Autodesk Fusion 360 part; units mm, degrees
(part 30 of 40)
  line L6927 (266.9246, 183.2292) -> (267.0281, 183.3491) construction
  line L6928 (267.0281, 183.3491) -> (267.1308, 183.47) construction
  line L6929 (267.1308, 183.47) -> (267.2327, 183.5919) construction
  line L6930 (267.2327, 183.5919) -> (267.3337, 183.7148) construction
  line L6931 (267.3337, 183.7148) -> (267.434, 183.8386) construction
  line L6932 (267.434, 183.8386) -> (267.5335, 183.9633) construction
  line L6933 (267.5335, 183.9633) -> (267.6323, 184.0888) construction
  line L6934 (267.6323, 184.0888) -> (267.7304, 184.2151) construction
  line L6935 (267.7304, 184.2151) -> (267.8277, 184.3423) construction
  line L6936 (267.8277, 184.3423) -> (267.9243, 184.4703) construction
  line L6937 (267.9243, 184.4703) -> (268.0201, 184.5991) construction
  line L6938 (268.0201, 184.5991) -> (268.1152, 184.7288) construction
  line L6939 (268.1152, 184.7288) -> (268.2096, 184.8592) construction
  line L6940 (268.2096, 184.8592) -> (268.3032, 184.9905) construction
  line L6941 (268.3032, 184.9905) -> (268.3962, 185.1224) construction
  line L6942 (268.3962, 185.1224) -> (268.4884, 185.2552) construction
  line L6943 (268.4884, 185.2552) -> (268.58, 185.3886) construction
  line L6944 (268.58, 185.3886) -> (268.6708, 185.5228) construction
  line L6945 (268.6708, 185.5228) -> (268.761, 185.6577) construction
  line L6946 (268.761, 185.6577) -> (268.8505, 185.7933) construction
  line L6947 (268.8505, 185.7933) -> (268.9393, 185.9295) construction
  line L6948 (268.9393, 185.9295) -> (269.0275, 186.0665) construction
  line L6949 (269.0275, 186.0665) -> (269.1149, 186.2042) construction
  line L6950 (269.1149, 186.2042) -> (269.2017, 186.3425) construction
  line L6951 (269.2017, 186.3425) -> (269.2878, 186.4815) construction
  line L6952 (269.2878, 186.4815) -> (269.3733, 186.6211) construction
  line L6953 (269.3733, 186.6211) -> (269.4581, 186.7614) construction
  line L6954 (269.4581, 186.7614) -> (269.5422, 186.9023) construction
  line L6955 (269.5422, 186.9023) -> (269.6257, 187.0438) construction
  line L6956 (269.6257, 187.0438) -> (269.7085, 187.186) construction
  line L6957 (269.7085, 187.186) -> (269.7907, 187.3288) construction
  line L6958 (269.7907, 187.3288) -> (269.8723, 187.4721) construction
  line L6959 (269.8723, 187.4721) -> (269.9532, 187.6161) construction
  line L6960 (269.9532, 187.6161) -> (270.0334, 187.7607) construction
  line L6961 (270.0334, 187.7607) -> (270.113, 187.9058) construction
  line L6962 (270.113, 187.9058) -> (270.192, 188.0515) construction
  line L6963 (270.192, 188.0515) -> (270.2703, 188.1978) construction
  line L6964 (270.2703, 188.1978) -> (270.348, 188.3447) construction
  line L6965 (270.348, 188.3447) -> (270.4251, 188.4921) construction
  line L6966 (270.4251, 188.4921) -> (270.5015, 188.6401) construction
  line L6967 (270.5015, 188.6401) -> (270.5773, 188.7886) construction
  line L6968 (270.5773, 188.7886) -> (270.6525, 188.9377) construction
  line L6969 (270.6525, 188.9377) -> (270.727, 189.0873) construction
  line L6970 (270.727, 189.0873) -> (270.801, 189.2374) construction
  line L6971 (270.801, 189.2374) -> (270.8743, 189.3881) construction
  line L6972 (270.8743, 189.3881) -> (270.9469, 189.5393) construction
  line L6973 (270.9469, 189.5393) -> (271.019, 189.6909) construction
  line L6974 (271.019, 189.6909) -> (271.0904, 189.8431) construction
  line L6975 (271.0904, 189.8431) -> (271.1471, 189.9653) construction
  line L6976 (271.1471, 189.9653) -> (271.1893, 190.0572) construction
  line L6977 (271.1893, 190.0572) -> (271.2173, 190.1185) construction
  line L6978 (271.2173, 190.1185) -> (271.2313, 190.1492) construction
  arc A182 (271.2762, 144.4572) -> (269.1057, 142.7194) centre (271.0895, 142.4659) ccw
  spline S93 degree 5 poles (264.6423, 118.8885) (264.6688, 118.8728) (264.7215, 118.8406) (264.7992, 118.7903) (264.9001, 118.7193) (265.0226, 118.6252) (265.1426, 118.5273) (265.2609, 118.4271) (265.3784, 118.3256) (265.4954, 118.2233) (265.6117, 118.12) (265.7271, 118.0156) (265.8414, 117.9097) (265.9544, 117.8019) (266.066, 117.6923) (266.1764, 117.581) (266.2857, 117.4684) (266.3942, 117.3545) (266.5018, 117.2397) (266.6087, 117.124) (266.7148, 117.0073) (266.8201, 116.8895) (266.9246, 116.7708) (267.0281, 116.6509) (267.1308, 116.53) (267.2327, 116.4081) (267.3337, 116.2852) (267.434, 116.1614) (267.5335, 116.0367) (267.6323, 115.9112) (267.7304, 115.7849) (267.8277, 115.6577) (267.9243, 115.5297) (268.0201, 115.4009) (268.1152, 115.2712) (268.2096, 115.1408) (268.3032, 115.0095) (268.3962, 114.8776) (268.4884, 114.7448) (268.58, 114.6114) (268.6708, 114.4772) (268.761, 114.3423) (268.8505, 114.2067) (268.9393, 114.0705) (269.0275, 113.9335) (269.1149, 113.7958) (269.2017, 113.6575) (269.2878, 113.5185) (269.3733, 113.3789) (269.4581, 113.2386) (269.5422, 113.0977) (269.6257, 112.9562) (269.7085, 112.814) (269.7907, 112.6712) (269.8723, 112.5279) (269.9532, 112.3839) (270.0334, 112.2393) (270.113, 112.0942) (270.192, 111.9485) (270.2703, 111.8022) (270.348, 111.6553) (270.4251, 111.5079) (270.5015, 111.3599) (270.5773, 111.2114) (270.6525, 111.0623) (270.727, 110.9127) (270.801, 110.7626) (270.8743, 110.6119) (270.9469, 110.4607) (271.019, 110.3091) (271.0904, 110.1569) (271.1471, 110.0347) (271.1893, 109.9428) (271.2173, 109.8815) (271.2313, 109.8508) knots 0 0 0 0 0 0 0.01428571 0.02857143 0.04285714 0.05714286 0.07142857 0.08571429 0.1 0.11428571 0.12857143 0.14285714 0.15714286 0.17142857 0.18571429 0.2 0.21428571 0.22857143 0.24285714 0.25714286 0.27142857 0.28571429 0.3 0.31428571 0.32857143 0.34285714 0.35714286 0.37142857 0.38571429 0.4 0.41428571 0.42857143 0.44285714 0.45714286 0.47142857 0.48571429 0.5 0.51428571 0.52857143 0.54285714 0.55714286 0.57142857 0.58571429 0.6 0.61428571 0.62857143 0.64285714 0.65714286 0.67142857 0.68571429 0.7 0.71428571 0.72857143 0.74285714 0.75714286 0.77142857 0.78571429 0.8 0.81428571 0.82857143 0.84285714 0.85714286 0.87142857 0.88571429 0.9 0.91428571 0.92857143 0.94285714 0.95714286 0.97142857 0.98571429 1 1 1 1 1 1
  line L6979 (264.6423, 118.8885) -> (264.6688, 118.8728) construction
  line L6980 (264.6688, 118.8728) -> (264.7215, 118.8406) construction
  line L6981 (264.7215, 118.8406) -> (264.7992, 118.7903) construction
  line L6982 (264.7992, 118.7903) -> (264.9001, 118.7193) construction
  line L6983 (264.9001, 118.7193) -> (265.0226, 118.6252) construction
  line L6984 (265.0226, 118.6252) -> (265.1426, 118.5273) construction
  line L6985 (265.1426, 118.5273) -> (265.2609, 118.4271) construction
  line L6986 (265.2609, 118.4271) -> (265.3784, 118.3256) construction
  line L6987 (265.3784, 118.3256) -> (265.4954, 118.2233) construction
  line L6988 (265.4954, 118.2233) -> (265.6117, 118.12) construction
  line L6989 (265.6117, 118.12) -> (265.7271, 118.0156) construction
  line L6990 (265.7271, 118.0156) -> (265.8414, 117.9097) construction
  line L6991 (265.8414, 117.9097) -> (265.9544, 117.8019) construction
  line L6992 (265.9544, 117.8019) -> (266.066, 117.6923) construction
  line L6993 (266.066, 117.6923) -> (266.1764, 117.581) construction
  line L6994 (266.1764, 117.581) -> (266.2857, 117.4684) construction
  line L6995 (266.2857, 117.4684) -> (266.3942, 117.3545) construction
  line L6996 (266.3942, 117.3545) -> (266.5018, 117.2397) construction
  line L6997 (266.5018, 117.2397) -> (266.6087, 117.124) construction
  line L6998 (266.6087, 117.124) -> (266.7148, 117.0073) construction
  line L6999 (266.7148, 117.0073) -> (266.8201, 116.8895) construction
  line L7000 (266.8201, 116.8895) -> (266.9246, 116.7708) construction
  line L7001 (266.9246, 116.7708) -> (267.0281, 116.6509) construction
  line L7002 (267.0281, 116.6509) -> (267.1308, 116.53) construction
  line L7003 (267.1308, 116.53) -> (267.2327, 116.4081) construction
  line L7004 (267.2327, 116.4081) -> (267.3337, 116.2852) construction
  line L7005 (267.3337, 116.2852) -> (267.434, 116.1614) construction
  line L7006 (267.434, 116.1614) -> (267.5335, 116.0367) construction
  line L7007 (267.5335, 116.0367) -> (267.6323, 115.9112) construction
  line L7008 (267.6323, 115.9112) -> (267.7304, 115.7849) construction
  line L7009 (267.7304, 115.7849) -> (267.8277, 115.6577) construction
  line L7010 (267.8277, 115.6577) -> (267.9243, 115.5297) construction
  line L7011 (267.9243, 115.5297) -> (268.0201, 115.4009) construction
  line L7012 (268.0201, 115.4009) -> (268.1152, 115.2712) construction
  line L7013 (268.1152, 115.2712) -> (268.2096, 115.1408) construction
  line L7014 (268.2096, 115.1408) -> (268.3032, 115.0095) construction
  line L7015 (268.3032, 115.0095) -> (268.3962, 114.8776) construction
  line L7016 (268.3962, 114.8776) -> (268.4884, 114.7448) construction
  line L7017 (268.4884, 114.7448) -> (268.58, 114.6114) construction
  line L7018 (268.58, 114.6114) -> (268.6708, 114.4772) construction
  line L7019 (268.6708, 114.4772) -> (268.761, 114.3423) construction
  line L7020 (268.761, 114.3423) -> (268.8505, 114.2067) construction
  line L7021 (268.8505, 114.2067) -> (268.9393, 114.0705) construction
  line L7022 (268.9393, 114.0705) -> (269.0275, 113.9335) construction
  line L7023 (269.0275, 113.9335) -> (269.1149, 113.7958) construction
  line L7024 (269.1149, 113.7958) -> (269.2017, 113.6575) construction
  line L7025 (269.2017, 113.6575) -> (269.2878, 113.5185) construction
  line L7026 (269.2878, 113.5185) -> (269.3733, 113.3789) construction
  line L7027 (269.3733, 113.3789) -> (269.4581, 113.2386) construction
  line L7028 (269.4581, 113.2386) -> (269.5422, 113.0977) construction
  line L7029 (269.5422, 113.0977) -> (269.6257, 112.9562) construction
  line L7030 (269.6257, 112.9562) -> (269.7085, 112.814) construction
  line L7031 (269.7085, 112.814) -> (269.7907, 112.6712) construction
  line L7032 (269.7907, 112.6712) -> (269.8723, 112.5279) construction
  line L7033 (269.8723, 112.5279) -> (269.9532, 112.3839) construction
  line L7034 (269.9532, 112.3839) -> (270.0334, 112.2393) construction
  line L7035 (270.0334, 112.2393) -> (270.113, 112.0942) construction
  line L7036 (270.113, 112.0942) -> (270.192, 111.9485) construction
  line L7037 (270.192, 111.9485) -> (270.2703, 111.8022) construction
  line L7038 (270.2703, 111.8022) -> (270.348, 111.6553) construction
  line L7039 (270.348, 111.6553) -> (270.4251, 111.5079) construction
  line L7040 (270.4251, 111.5079) -> (270.5015, 111.3599) construction
  line L7041 (270.5015, 111.3599) -> (270.5773, 111.2114) construction
  line L7042 (270.5773, 111.2114) -> (270.6525, 111.0623) construction
  line L7043 (270.6525, 111.0623) -> (270.727, 110.9127) construction
  line L7044 (270.727, 110.9127) -> (270.801, 110.7626) construction
  line L7045 (270.801, 110.7626) -> (270.8743, 110.6119) construction
  line L7046 (270.8743, 110.6119) -> (270.9469, 110.4607) construction
  line L7047 (270.9469, 110.4607) -> (271.019, 110.3091) construction
  line L7048 (271.019, 110.3091) -> (271.0904, 110.1569) construction
  line L7049 (271.0904, 110.1569) -> (271.1471, 110.0347) construction
  line L7050 (271.1471, 110.0347) -> (271.1893, 109.9428) construction
  line L7051 (271.1893, 109.9428) -> (271.2173, 109.8815) construction
  line L7052 (271.2173, 109.8815) -> (271.2313, 109.8508) construction
  line L7053 (188.5839, 95.4634) -> (187.9372, 93.9655)
  line L7054 (161.0254, 180.2798) -> (159.6217, 181.1115)
  spline S94 degree 5 poles (151.3635, 155.6951) (151.3327, 155.6979) (151.2711, 155.7029) (151.1787, 155.7078) (151.0554, 155.7097) (150.901, 155.7056) (150.7464, 155.6969) (150.5917, 155.6854) (150.437, 155.6723) (150.2822, 155.6583) (150.1275, 155.6431) (149.9727, 155.6265) (149.818, 155.608) (149.6632, 155.5871) (149.5085, 155.5641) (149.3538, 155.539) (149.1991, 155.5121) (149.0445, 155.4838) (148.8899, 155.4542) (148.7354, 155.4233) (148.5809, 155.3913) (148.4265, 155.3579) (148.2722, 155.3232) (148.118, 155.2871) (147.9638, 155.2497) (147.8098, 155.2109) (147.6558, 155.1709) (147.5019, 155.1297) (147.3481, 155.0873) (147.1944, 155.0439) (147.0408, 154.9993) (146.8873, 154.9536) (146.734, 154.9068) (146.5807, 154.8589) (146.4276, 154.8099) (146.2746, 154.7599) (146.1217, 154.7087) (145.9689, 154.6566) (145.8162, 154.6035) (145.6637, 154.5493) (145.5114, 154.4942) (145.3591, 154.438) (145.207, 154.381) (145.055, 154.3229) (144.9032, 154.2639) (144.7516, 154.2039) (144.6, 154.143) (144.4487, 154.0812) (144.2975, 154.0185) (144.1464, 153.9548) (143.9955, 153.8903) (143.8448, 153.8249) (143.6942, 153.7585) (143.5438, 153.6913) (143.3936, 153.6233) (143.2435, 153.5543) (143.0936, 153.4846) (142.9439, 153.4139) (142.7944, 153.3425) (142.645, 153.2701) (142.4958, 153.197) (142.3468, 153.123) (142.198, 153.0482) (142.0494, 152.9726) (141.9009, 152.8962) (141.7527, 152.819) (141.6046, 152.741) (141.4568, 152.6622) (141.3091, 152.5826) (141.1617, 152.5023) (141.0144, 152.4211) (140.8968, 152.3556) (140.8086, 152.3061) (140.7499, 152.2729) (140.7205, 152.2563) knots 0 0 0 0 0 0 0.01428571 0.02857143 0.04285714 0.05714286 0.07142857 0.08571429 0.1 0.11428571 0.12857143 0.14285714 0.15714286 0.17142857 0.18571429 0.2 0.21428571 0.22857143 0.24285714 0.25714286 0.27142857 0.28571429 0.3 0.31428571 0.32857143 0.34285714 0.35714286 0.37142857 0.38571429 0.4 0.41428571 0.42857143 0.44285714 0.45714286 0.47142857 0.48571429 0.5 0.51428571 0.52857143 0.54285714 0.55714286 0.57142857 0.58571429 0.6 0.61428571 0.62857143 0.64285714 0.65714286 0.67142857 0.68571429 0.7 0.71428571 0.72857143 0.74285714 0.75714286 0.77142857 0.78571429 0.8 0.81428571 0.82857143 0.84285714 0.85714286 0.87142857 0.88571429 0.9 0.91428571 0.92857143 0.94285714 0.95714286 0.97142857 0.98571429 1 1 1 1 1 1
  line L7055 (151.3635, 155.6951) -> (151.3327, 155.6979) construction
  line L7056 (151.3327, 155.6979) -> (151.2711, 155.7029) construction
  line L7057 (151.2711, 155.7029) -> (151.1787, 155.7078) construction
  line L7058 (151.1787, 155.7078) -> (151.0554, 155.7097) construction
  line L7059 (151.0554, 155.7097) -> (150.901, 155.7056) construction
  line L7060 (150.901, 155.7056) -> (150.7464, 155.6969) construction
  line L7061 (150.7464, 155.6969) -> (150.5917, 155.6854) construction
  line L7062 (150.5917, 155.6854) -> (150.437, 155.6723) construction
  line L7063 (150.437, 155.6723) -> (150.2822, 155.6583) construction
  line L7064 (150.2822, 155.6583) -> (150.1275, 155.6431) construction
  line L7065 (150.1275, 155.6431) -> (149.9727, 155.6265) construction
  line L7066 (149.9727, 155.6265) -> (149.818, 155.608) construction
  line L7067 (149.818, 155.608) -> (149.6632, 155.5871) construction
  line L7068 (149.6632, 155.5871) -> (149.5085, 155.5641) construction
  line L7069 (149.5085, 155.5641) -> (149.3538, 155.539) construction
  line L7070 (149.3538, 155.539) -> (149.1991, 155.5121) construction
  line L7071 (149.1991, 155.5121) -> (149.0445, 155.4838) construction
  line L7072 (149.0445, 155.4838) -> (148.8899, 155.4542) construction
  line L7073 (148.8899, 155.4542) -> (148.7354, 155.4233) construction
  line L7074 (148.7354, 155.4233) -> (148.5809, 155.3913) construction
  line L7075 (148.5809, 155.3913) -> (148.4265, 155.3579) construction
  line L7076 (148.4265, 155.3579) -> (148.2722, 155.3232) construction
  line L7077 (148.2722, 155.3232) -> (148.118, 155.2871) construction
  line L7078 (148.118, 155.2871) -> (147.9638, 155.2497) construction
  line L7079 (147.9638, 155.2497) -> (147.8098, 155.2109) construction
  line L7080 (147.8098, 155.2109) -> (147.6558, 155.1709) construction
  line L7081 (147.6558, 155.1709) -> (147.5019, 155.1297) construction
  line L7082 (147.5019, 155.1297) -> (147.3481, 155.0873) construction
  line L7083 (147.3481, 155.0873) -> (147.1944, 155.0439) construction
  line L7084 (147.1944, 155.0439) -> (147.0408, 154.9993) construction
  line L7085 (147.0408, 154.9993) -> (146.8873, 154.9536) construction
  line L7086 (146.8873, 154.9536) -> (146.734, 154.9068) construction
  line L7087 (146.734, 154.9068) -> (146.5807, 154.8589) construction
  line L7088 (146.5807, 154.8589) -> (146.4276, 154.8099) construction
  line L7089 (146.4276, 154.8099) -> (146.2746, 154.7599) construction
  line L7090 (146.2746, 154.7599) -> (146.1217, 154.7087) construction
  line L7091 (146.1217, 154.7087) -> (145.9689, 154.6566) construction
  line L7092 (145.9689, 154.6566) -> (145.8162, 154.6035) construction
  line L7093 (145.8162, 154.6035) -> (145.6637, 154.5493) construction
  line L7094 (145.6637, 154.5493) -> (145.5114, 154.4942) construction
  line L7095 (145.5114, 154.4942) -> (145.3591, 154.438) construction
  line L7096 (145.3591, 154.438) -> (145.207, 154.381) construction
  line L7097 (145.207, 154.381) -> (145.055, 154.3229) construction
  line L7098 (145.055, 154.3229) -> (144.9032, 154.2639) construction
  line L7099 (144.9032, 154.2639) -> (144.7516, 154.2039) construction
  line L7100 (144.7516, 154.2039) -> (144.6, 154.143) construction
  line L7101 (144.6, 154.143) -> (144.4487, 154.0812) construction
  line L7102 (144.4487, 154.0812) -> (144.2975, 154.0185) construction
  line L7103 (144.2975, 154.0185) -> (144.1464, 153.9548) construction
  line L7104 (144.1464, 153.9548) -> (143.9955, 153.8903) construction
  line L7105 (143.9955, 153.8903) -> (143.8448, 153.8249) construction
  line L7106 (143.8448, 153.8249) -> (143.6942, 153.7585) construction
  line L7107 (143.6942, 153.7585) -> (143.5438, 153.6913) construction
  line L7108 (143.5438, 153.6913) -> (143.3936, 153.6233) construction
  line L7109 (143.3936, 153.6233) -> (143.2435, 153.5543) construction
  line L7110 (143.2435, 153.5543) -> (143.0936, 153.4846) construction
  line L7111 (143.0936, 153.4846) -> (142.9439, 153.4139) construction
  line L7112 (142.9439, 153.4139) -> (142.7944, 153.3425) construction
  line L7113 (142.7944, 153.3425) -> (142.645, 153.2701) construction
  line L7114 (142.645, 153.2701) -> (142.4958, 153.197) construction
  line L7115 (142.4958, 153.197) -> (142.3468, 153.123) construction
  line L7116 (142.3468, 153.123) -> (142.198, 153.0482) construction
  line L7117 (142.198, 153.0482) -> (142.0494, 152.9726) construction
  line L7118 (142.0494, 152.9726) -> (141.9009, 152.8962) construction
  line L7119 (141.9009, 152.8962) -> (141.7527, 152.819) construction
  line L7120 (141.7527, 152.819) -> (141.6046, 152.741) construction
  line L7121 (141.6046, 152.741) -> (141.4568, 152.6622) construction
  line L7122 (141.4568, 152.6622) -> (141.3091, 152.5826) construction
  line L7123 (141.3091, 152.5826) -> (141.1617, 152.5023) construction
  line L7124 (141.1617, 152.5023) -> (141.0144, 152.4211) construction
  line L7125 (141.0144, 152.4211) -> (140.8968, 152.3556) construction
  line L7126 (140.8968, 152.3556) -> (140.8086, 152.3061) construction
  line L7127 (140.8086, 152.3061) -> (140.7499, 152.2729) construction
  line L7128 (140.7499, 152.2729) -> (140.7205, 152.2563) construction
  line L7129 (167.5414, 189.2483) -> (166.3167, 190.3263)
  line L7130 (172.8837, 194.5906) -> (171.8057, 195.8153)
  line L7131 (242.4118, 201.1066) -> (243.2435, 202.5103)
  line L7132 (263.2386, 180.2798) -> (264.6423, 181.1115)
  line L7133 (251.3803, 105.4094) -> (252.4583, 104.1847)
  line L7134 (206.5892, 90.8558) -> (206.4369, 89.2315)
  line L7135 (251.3803, 105.4094) -> (252.4583, 104.1847)
  line L7136 (199.127, 92.0377) -> (198.7698, 90.4458)
  line L7137 (181.8522, 98.8934) -> (181.0205, 97.4897)
  arc A183 (206.5892, 90.8558) -> (204.8514, 93.0263) centre (204.5979, 91.0425) ccw
  arc A184 (154.1697, 136.995) -> (155.697, 139.3184) centre (153.7319, 138.9465) ccw
  arc A185 (235.6801, 204.5366) -> (236.6621, 201.9354) centre (237.5162, 203.7438) ccw
  spline S95 degree 5 poles (187.9372, 93.9655) (187.9249, 93.9372) (187.9012, 93.8802) (187.868, 93.7938) (187.8281, 93.6771) (187.7842, 93.5289) (187.7447, 93.3792) (187.7079, 93.2286) (187.6725, 93.0774) (187.638, 92.9259) (187.6046, 92.774) (187.5726, 92.6217) (187.5424, 92.4688) (187.5144, 92.3152) (187.4885, 92.1609) (187.4646, 92.006) (187.4423, 91.8506) (187.4215, 91.6948) (187.4019, 91.5386) (187.3835, 91.3821) (187.3662, 91.2253) (187.3502, 91.0682) (187.3355, 90.9107) (187.3222, 90.7529) (187.3102, 90.5947) (187.2995, 90.4362) (187.29, 90.2774) (187.2816, 90.1183) (187.2743, 89.9589) (187.2682, 89.7993) (187.2631, 89.6395) (187.2591, 89.4794) (187.2563, 89.3191) (187.2544, 89.1585) (187.2537, 88.9977) (187.254, 88.8367) (187.2554, 88.6755) (187.2578, 88.5141) (187.2612, 88.3525) (187.2655, 88.1907) (187.2709, 88.0288) (187.2772, 87.8666) (187.2845, 87.7043) (187.2928, 87.5419) (187.302, 87.3793) (187.3121, 87.2165) (187.3232, 87.0536) (187.3353, 86.8905) (187.3482, 86.7273) (187.362, 86.564) (187.3768, 86.4005) (187.3924, 86.2369) (187.409, 86.0732) (187.4264, 85.9094) (187.4447, 85.7455) (187.4639, 85.5815) (187.484, 85.4174) (187.5049, 85.2532) (187.5266, 85.0889) (187.5492, 84.9245) (187.5727, 84.76) (187.597, 84.5954) (187.6222, 84.4308) (187.6481, 84.266) (187.6749, 84.1013) (187.7026, 83.9364) (187.731, 83.7715) (187.7602, 83.6065) (187.7903, 83.4415) (187.8212, 83.2764) (187.8528, 83.1113) (187.8788, 82.9792) (187.8986, 82.8801) (187.912, 82.814) (187.9188, 82.7809) knots 0 0 0 0 0 0 0.01428571 0.02857143 0.04285714 0.05714286 0.07142857 0.08571429 0.1 0.11428571 0.12857143 0.14285714 0.15714286 0.17142857 0.18571429 0.2 0.21428571 0.22857143 0.24285714 0.25714286 0.27142857 0.28571429 0.3 0.31428571 0.32857143 0.34285714 0.35714286 0.37142857 0.38571429 0.4 0.41428571 0.42857143 0.44285714 0.45714286 0.47142857 0.48571429 0.5 0.51428571 0.52857143 0.54285714 0.55714286 0.57142857 0.58571429 0.6 0.61428571 0.62857143 0.64285714 0.65714286 0.67142857 0.68571429 0.7 0.71428571 0.72857143 0.74285714 0.75714286 0.77142857 0.78571429 0.8 0.81428571 0.82857143 0.84285714 0.85714286 0.87142857 0.88571429 0.9 0.91428571 0.92857143 0.94285714 0.95714286 0.97142857 0.98571429 1 1 1 1 1 1
  line L7138 (187.9372, 93.9655) -> (187.9249, 93.9372) construction
  line L7139 (187.9249, 93.9372) -> (187.9012, 93.8802) construction
  line L7140 (187.9012, 93.8802) -> (187.868, 93.7938) construction
  line L7141 (187.868, 93.7938) -> (187.8281, 93.6771) construction
  line L7142 (187.8281, 93.6771) -> (187.7842, 93.5289) construction
  line L7143 (187.7842, 93.5289) -> (187.7447, 93.3792) construction
  line L7144 (187.7447, 93.3792) -> (187.7079, 93.2286) construction
  line L7145 (187.7079, 93.2286) -> (187.6725, 93.0774) construction
  line L7146 (187.6725, 93.0774) -> (187.638, 92.9259) construction
  line L7147 (187.638, 92.9259) -> (187.6046, 92.774) construction
  line L7148 (187.6046, 92.774) -> (187.5726, 92.6217) construction
  line L7149 (187.5726, 92.6217) -> (187.5424, 92.4688) construction
  line L7150 (187.5424, 92.4688) -> (187.5144, 92.3152) construction
  line L7151 (187.5144, 92.3152) -> (187.4885, 92.1609) construction
  line L7152 (187.4885, 92.1609) -> (187.4646, 92.006) construction
  line L7153 (187.4646, 92.006) -> (187.4423, 91.8506) construction
  line L7154 (187.4423, 91.8506) -> (187.4215, 91.6948) construction
  line L7155 (187.4215, 91.6948) -> (187.4019, 91.5386) construction
  line L7156 (187.4019, 91.5386) -> (187.3835, 91.3821) construction
  line L7157 (187.3835, 91.3821) -> (187.3662, 91.2253) construction
  line L7158 (187.3662, 91.2253) -> (187.3502, 91.0682) construction
  line L7159 (187.3502, 91.0682) -> (187.3355, 90.9107) construction
  line L7160 (187.3355, 90.9107) -> (187.3222, 90.7529) construction
  line L7161 (187.3222, 90.7529) -> (187.3102, 90.5947) construction
  line L7162 (187.3102, 90.5947) -> (187.2995, 90.4362) construction
  line L7163 (187.2995, 90.4362) -> (187.29, 90.2774) construction
  line L7164 (187.29, 90.2774) -> (187.2816, 90.1183) construction
  line L7165 (187.2816, 90.1183) -> (187.2743, 89.9589) construction
  line L7166 (187.2743, 89.9589) -> (187.2682, 89.7993) construction
  line L7167 (187.2682, 89.7993) -> (187.2631, 89.6395) construction
  line L7168 (187.2631, 89.6395) -> (187.2591, 89.4794) construction
  line L7169 (187.2591, 89.4794) -> (187.2563, 89.3191) construction
  line L7170 (187.2563, 89.3191) -> (187.2544, 89.1585) construction
  line L7171 (187.2544, 89.1585) -> (187.2537, 88.9977) construction
  line L7172 (187.2537, 88.9977) -> (187.254, 88.8367) construction
  line L7173 (187.254, 88.8367) -> (187.2554, 88.6755) construction
  line L7174 (187.2554, 88.6755) -> (187.2578, 88.5141) construction
  line L7175 (187.2578, 88.5141) -> (187.2612, 88.3525) construction
  line L7176 (187.2612, 88.3525) -> (187.2655, 88.1907) construction
  line L7177 (187.2655, 88.1907) -> (187.2709, 88.0288) construction
  line L7178 (187.2709, 88.0288) -> (187.2772, 87.8666) construction
  line L7179 (187.2772, 87.8666) -> (187.2845, 87.7043) construction
  line L7180 (187.2845, 87.7043) -> (187.2928, 87.5419) construction
  line L7181 (187.2928, 87.5419) -> (187.302, 87.3793) construction
  line L7182 (187.302, 87.3793) -> (187.3121, 87.2165) construction
  line L7183 (187.3121, 87.2165) -> (187.3232, 87.0536) construction
  line L7184 (187.3232, 87.0536) -> (187.3353, 86.8905) construction
  line L7185 (187.3353, 86.8905) -> (187.3482, 86.7273) construction
  line L7186 (187.3482, 86.7273) -> (187.362, 86.564) construction
  line L7187 (187.362, 86.564) -> (187.3768, 86.4005) construction
  line L7188 (187.3768, 86.4005) -> (187.3924, 86.2369) construction
  line L7189 (187.3924, 86.2369) -> (187.409, 86.0732) construction
  line L7190 (187.409, 86.0732) -> (187.4264, 85.9094) construction
  line L7191 (187.4264, 85.9094) -> (187.4447, 85.7455) construction
  line L7192 (187.4447, 85.7455) -> (187.4639, 85.5815) construction
  line L7193 (187.4639, 85.5815) -> (187.484, 85.4174) construction
  line L7194 (187.484, 85.4174) -> (187.5049, 85.2532) construction
  line L7195 (187.5049, 85.2532) -> (187.5266, 85.0889) construction
  line L7196 (187.5266, 85.0889) -> (187.5492, 84.9245) construction
  line L7197 (187.5492, 84.9245) -> (187.5727, 84.76) construction
  line L7198 (187.5727, 84.76) -> (187.597, 84.5954) construction
  line L7199 (187.597, 84.5954) -> (187.6222, 84.4308) construction
  line L7200 (187.6222, 84.4308) -> (187.6481, 84.266) construction
  line L7201 (187.6481, 84.266) -> (187.6749, 84.1013) construction
  line L7202 (187.6749, 84.1013) -> (187.7026, 83.9364) construction
  line L7203 (187.7026, 83.9364) -> (187.731, 83.7715) construction
  line L7204 (187.731, 83.7715) -> (187.7602, 83.6065) construction
  line L7205 (187.7602, 83.6065) -> (187.7903, 83.4415) construction
  line L7206 (187.7903, 83.4415) -> (187.8212, 83.2764) construction
  line L7207 (187.8212, 83.2764) -> (187.8528, 83.1113) construction
  line L7208 (187.8528, 83.1113) -> (187.8788, 82.9792) construction
  line L7209 (187.8788, 82.9792) -> (187.8986, 82.8801) construction
  line L7210 (187.8986, 82.8801) -> (187.912, 82.814) construction
  line L7211 (187.912, 82.814) -> (187.9188, 82.7809) construction
  arc A186 (168.332, 93.5531) -> (171.9828, 90.9007) centre (212.132, 150) ccw
  arc A187 (192.2105, 218.6136) -> (187.9188, 217.2191) centre (212.132, 150) ccw
  spline S96 degree 5 poles (217.8271, 210.7685) (217.8299, 210.7993) (217.8349, 210.8609) (217.8398, 210.9533) (217.8417, 211.0766) (217.8376, 211.231) (217.8289, 211.3856) (217.8174, 211.5403) (217.8043, 211.695) (217.7903, 211.8498) (217.7751, 212.0045) (217.7585, 212.1593) (217.74, 212.314) (217.7191, 212.4688) (217.6961, 212.6235) (217.671, 212.7782) (217.6441, 212.9329) (217.6158, 213.0875) (217.5862, 213.2421) (217.5553, 213.3966) (217.5233, 213.5511) (217.4899, 213.7055) (217.4552, 213.8598) (217.4191, 214.014) (217.3817, 214.1682) (217.3429, 214.3222) (217.3029, 214.4762) (217.2617, 214.6301) (217.2193, 214.7839) (217.1759, 214.9376) (217.1313, 215.0912) (217.0856, 215.2447) (217.0388, 215.398) (216.9909, 215.5513) (216.9419, 215.7044) (216.8919, 215.8574) (216.8407, 216.0103) (216.7886, 216.1631) (216.7355, 216.3158) (216.6813, 216.4683) (216.6262, 216.6206) (216.57, 216.7729) (216.513, 216.925) (216.4549, 217.077) (216.3959, 217.2288) (216.3359, 217.3804) (216.275, 217.532) (216.2132, 217.6833) (216.1505, 217.8345) (216.0868, 217.9856) (216.0223, 218.1365) (215.9569, 218.2872) (215.8905, 218.4378) (215.8233, 218.5882) (215.7553, 218.7384) (215.6863, 218.8885) (215.6166, 219.0384) (215.5459, 219.1881) (215.4745, 219.3376) (215.4021, 219.487) (215.329, 219.6362) (215.255, 219.7852) (215.1802, 219.934) (215.1046, 220.0826) (215.0282, 220.2311) (214.951, 220.3793) (214.873, 220.5274) (214.7942, 220.6752) (214.7146, 220.8229) (214.6343, 220.9703) (214.5531, 221.1176) (214.4876, 221.2352) (214.4381, 221.3234) (214.4049, 221.3821) (214.3883, 221.4115) knots 0 0 0 0 0 0 0.01428571 0.02857143 0.04285714 0.05714286 0.07142857 0.08571429 0.1 0.11428571 0.12857143 0.14285714 0.15714286 0.17142857 0.18571429 0.2 0.21428571 0.22857143 0.24285714 0.25714286 0.27142857 0.28571429 0.3 0.31428571 0.32857143 0.34285714 0.35714286 0.37142857 0.38571429 0.4 0.41428571 0.42857143 0.44285714 0.45714286 0.47142857 0.48571429 0.5 0.51428571 0.52857143 0.54285714 0.55714286 0.57142857 0.58571429 0.6 0.61428571 0.62857143 0.64285714 0.65714286 0.67142857 0.68571429 0.7 0.71428571 0.72857143 0.74285714 0.75714286 0.77142857 0.78571429 0.8 0.81428571 0.82857143 0.84285714 0.85714286 0.87142857 0.88571429 0.9 0.91428571 0.92857143 0.94285714 0.95714286 0.97142857 0.98571429 1 1 1 1 1 1
  line L7212 (217.8271, 210.7685) -> (217.8299, 210.7993) construction
  line L7213 (217.8299, 210.7993) -> (217.8349, 210.8609) construction
  line L7214 (217.8349, 210.8609) -> (217.8398, 210.9533) construction
  line L7215 (217.8398, 210.9533) -> (217.8417, 211.0766) construction
  line L7216 (217.8417, 211.0766) -> (217.8376, 211.231) construction
  line L7217 (217.8376, 211.231) -> (217.8289, 211.3856) construction
  line L7218 (217.8289, 211.3856) -> (217.8174, 211.5403) construction
  line L7219 (217.8174, 211.5403) -> (217.8043, 211.695) construction
  line L7220 (217.8043, 211.695) -> (217.7903, 211.8498) construction
  line L7221 (217.7903, 211.8498) -> (217.7751, 212.0045) construction
  line L7222 (217.7751, 212.0045) -> (217.7585, 212.1593) construction
  line L7223 (217.7585, 212.1593) -> (217.74, 212.314) construction
  line L7224 (217.74, 212.314) -> (217.7191, 212.4688) construction
  line L7225 (217.7191, 212.4688) -> (217.6961, 212.6235) construction
  line L7226 (217.6961, 212.6235) -> (217.671, 212.7782) construction
  line L7227 (217.671, 212.7782) -> (217.6441, 212.9329) construction
  line L7228 (217.6441, 212.9329) -> (217.6158, 213.0875) construction
  line L7229 (217.6158, 213.0875) -> (217.5862, 213.2421) construction
  line L7230 (217.5862, 213.2421) -> (217.5553, 213.3966) construction
  line L7231 (217.5553, 213.3966) -> (217.5233, 213.5511) construction
  line L7232 (217.5233, 213.5511) -> (217.4899, 213.7055) construction
  line L7233 (217.4899, 213.7055) -> (217.4552, 213.8598) construction
  line L7234 (217.4552, 213.8598) -> (217.4191, 214.014) construction
  line L7235 (217.4191, 214.014) -> (217.3817, 214.1682) construction
  line L7236 (217.3817, 214.1682) -> (217.3429, 214.3222) construction
  line L7237 (217.3429, 214.3222) -> (217.3029, 214.4762) construction
  line L7238 (217.3029, 214.4762) -> (217.2617, 214.6301) construction
  line L7239 (217.2617, 214.6301) -> (217.2193, 214.7839) construction
  line L7240 (217.2193, 214.7839) -> (217.1759, 214.9376) construction
  line L7241 (217.1759, 214.9376) -> (217.1313, 215.0912) construction
  line L7242 (217.1313, 215.0912) -> (217.0856, 215.2447) construction
  line L7243 (217.0856, 215.2447) -> (217.0388, 215.398) construction
  line L7244 (217.0388, 215.398) -> (216.9909, 215.5513) construction
  line L7245 (216.9909, 215.5513) -> (216.9419, 215.7044) construction
  line L7246 (216.9419, 215.7044) -> (216.8919, 215.8574) construction
  line L7247 (216.8919, 215.8574) -> (216.8407, 216.0103) construction
  line L7248 (216.8407, 216.0103) -> (216.7886, 216.1631) construction
  line L7249 (216.7886, 216.1631) -> (216.7355, 216.3158) construction
  line L7250 (216.7355, 216.3158) -> (216.6813, 216.4683) construction
  line L7251 (216.6813, 216.4683) -> (216.6262, 216.6206) construction
  line L7252 (216.6262, 216.6206) -> (216.57, 216.7729) construction
  line L7253 (216.57, 216.7729) -> (216.513, 216.925) construction
  line L7254 (216.513, 216.925) -> (216.4549, 217.077) construction
  line L7255 (216.4549, 217.077) -> (216.3959, 217.2288) construction
  line L7256 (216.3959, 217.2288) -> (216.3359, 217.3804) construction
  line L7257 (216.3359, 217.3804) -> (216.275, 217.532) construction
  line L7258 (216.275, 217.532) -> (216.2132, 217.6833) construction
  line L7259 (216.2132, 217.6833) -> (216.1505, 217.8345) construction
  line L7260 (216.1505, 217.8345) -> (216.0868, 217.9856) construction
  line L7261 (216.0868, 217.9856) -> (216.0223, 218.1365) construction
  line L7262 (216.0223, 218.1365) -> (215.9569, 218.2872) construction
  line L7263 (215.9569, 218.2872) -> (215.8905, 218.4378) construction
  line L7264 (215.8905, 218.4378) -> (215.8233, 218.5882) construction
  line L7265 (215.8233, 218.5882) -> (215.7553, 218.7384) construction
  line L7266 (215.7553, 218.7384) -> (215.6863, 218.8885) construction
  line L7267 (215.6863, 218.8885) -> (215.6166, 219.0384) construction
  line L7268 (215.6166, 219.0384) -> (215.5459, 219.1881) construction
  line L7269 (215.5459, 219.1881) -> (215.4745, 219.3376) construction
  line L7270 (215.4745, 219.3376) -> (215.4021, 219.487) construction
  line L7271 (215.4021, 219.487) -> (215.329, 219.6362) construction
  line L7272 (215.329, 219.6362) -> (215.255, 219.7852) construction
  line L7273 (215.255, 219.7852) -> (215.1802, 219.934) construction
  line L7274 (215.1802, 219.934) -> (215.1046, 220.0826) construction
  line L7275 (215.1046, 220.0826) -> (215.0282, 220.2311) construction
  line L7276 (215.0282, 220.2311) -> (214.951, 220.3793) construction
  line L7277 (214.951, 220.3793) -> (214.873, 220.5274) construction
  line L7278 (214.873, 220.5274) -> (214.7942, 220.6752) construction
  line L7279 (214.7942, 220.6752) -> (214.7146, 220.8229) construction
  line L7280 (214.7146, 220.8229) -> (214.6343, 220.9703) construction
  line L7281 (214.6343, 220.9703) -> (214.5531, 221.1176) construction
  line L7282 (214.5531, 221.1176) -> (214.4876, 221.2352) construction
  line L7283 (214.4876, 221.2352) -> (214.4381, 221.3234) construction
  line L7284 (214.4381, 221.3234) -> (214.4049, 221.3821) construction
  line L7285 (214.4049, 221.3821) -> (214.3883, 221.4115) construction
  spline S97 degree 5 poles (272.9005, 144.3049) (272.9313, 144.3021) (272.9929, 144.2971) (273.0853, 144.2922) (273.2086, 144.2903) (273.363, 144.2944) (273.5176, 144.3031) (273.6723, 144.3146) (273.827, 144.3277) (273.9818, 144.3417) (274.1365, 144.3569) (274.2913, 144.3735) (274.446, 144.392) (274.6008, 144.4129) (274.7555, 144.4359) (274.9102, 144.461) (275.0649, 144.4879) (275.2195, 144.5162) (275.3741, 144.5458) (275.5286, 144.5767) (275.6831, 144.6087) (275.8375, 144.6421) (275.9918, 144.6768) (276.146, 144.7129) (276.3002, 144.7503) (276.4542, 144.7891) (276.6082, 144.8291) (276.7621, 144.8703) (276.9159, 144.9127) (277.0696, 144.9561) (277.2232, 145.0007) (277.3767, 145.0464) (277.53, 145.0932) (277.6833, 145.1411) (277.8364, 145.1901) (277.9894, 145.2401) (278.1423, 145.2913) (278.2951, 145.3434) (278.4478, 145.3965) (278.6003, 145.4507) (278.7526, 145.5058) (278.9049, 145.562) (279.057, 145.619) (279.209, 145.6771) (279.3608, 145.7361) (279.5124, 145.7961) (279.664, 145.857) (279.8153, 145.9188) (279.9665, 145.9815) (280.1176, 146.0452) (280.2685, 146.1097) (280.4192, 146.1751) (280.5698, 146.2415) (280.7202, 146.3087) (280.8704, 146.3767) (281.0205, 146.4457) (281.1704, 146.5154) (281.3201, 146.5861) (281.4696, 146.6575) (281.619, 146.7299) (281.7682, 146.803) (281.9172, 146.877) (282.066, 146.9518) (282.2146, 147.0274) (282.3631, 147.1038) (282.5113, 147.181) (282.6594, 147.259) (282.8072, 147.3378) (282.9549, 147.4174) (283.1023, 147.4977) (283.2496, 147.5789) (283.3672, 147.6444) (283.4554, 147.6939) (283.5141, 147.7271) (283.5435, 147.7437) knots 0 0 0 0 0 0 0.01428571 0.02857143 0.04285714 0.05714286 0.07142857 0.08571429 0.1 0.11428571 0.12857143 0.14285714 0.15714286 0.17142857 0.18571429 0.2 0.21428571 0.22857143 0.24285714 0.25714286 0.27142857 0.28571429 0.3 0.31428571 0.32857143 0.34285714 0.35714286 0.37142857 0.38571429 0.4 0.41428571 0.42857143 0.44285714 0.45714286 0.47142857 0.48571429 0.5 0.51428571 0.52857143 0.54285714 0.55714286 0.57142857 0.58571429 0.6 0.61428571 0.62857143 0.64285714 0.65714286 0.67142857 0.68571429 0.7 0.71428571 0.72857143 0.74285714 0.75714286 0.77142857 0.78571429 0.8 0.81428571 0.82857143 0.84285714 0.85714286 0.87142857 0.88571429 0.9 0.91428571 0.92857143 0.94285714 0.95714286 0.97142857 0.98571429 1 1 1 1 1 1
  line L7286 (272.9005, 144.3049) -> (272.9313, 144.3021) construction
  line L7287 (272.9313, 144.3021) -> (272.9929, 144.2971) construction
  line L7288 (272.9929, 144.2971) -> (273.0853, 144.2922) construction
  line L7289 (273.0853, 144.2922) -> (273.2086, 144.2903) construction
  line L7290 (273.2086, 144.2903) -> (273.363, 144.2944) construction
  line L7291 (273.363, 144.2944) -> (273.5176, 144.3031) construction
  line L7292 (273.5176, 144.3031) -> (273.6723, 144.3146) construction
  line L7293 (273.6723, 144.3146) -> (273.827, 144.3277) construction
  line L7294 (273.827, 144.3277) -> (273.9818, 144.3417) construction
  line L7295 (273.9818, 144.3417) -> (274.1365, 144.3569) construction
  line L7296 (274.1365, 144.3569) -> (274.2913, 144.3735) construction
  line L7297 (274.2913, 144.3735) -> (274.446, 144.392) construction
  line L7298 (274.446, 144.392) -> (274.6008, 144.4129) construction
  line L7299 (274.6008, 144.4129) -> (274.7555, 144.4359) construction
  line L7300 (274.7555, 144.4359) -> (274.9102, 144.461) construction
  line L7301 (274.9102, 144.461) -> (275.0649, 144.4879) construction
  line L7302 (275.0649, 144.4879) -> (275.2195, 144.5162) construction
  line L7303 (275.2195, 144.5162) -> (275.3741, 144.5458) construction
  line L7304 (275.3741, 144.5458) -> (275.5286, 144.5767) construction
  line L7305 (275.5286, 144.5767) -> (275.6831, 144.6087) construction
  line L7306 (275.6831, 144.6087) -> (275.8375, 144.6421) construction
  line L7307 (275.8375, 144.6421) -> (275.9918, 144.6768) construction
  line L7308 (275.9918, 144.6768) -> (276.146, 144.7129) construction
  line L7309 (276.146, 144.7129) -> (276.3002, 144.7503) construction
  line L7310 (276.3002, 144.7503) -> (276.4542, 144.7891) construction
  line L7311 (276.4542, 144.7891) -> (276.6082, 144.8291) construction
  line L7312 (276.6082, 144.8291) -> (276.7621, 144.8703) construction
  line L7313 (276.7621, 144.8703) -> (276.9159, 144.9127) construction
  line L7314 (276.9159, 144.9127) -> (277.0696, 144.9561) construction
  line L7315 (277.0696, 144.9561) -> (277.2232, 145.0007) construction
  line L7316 (277.2232, 145.0007) -> (277.3767, 145.0464) construction
  line L7317 (277.3767, 145.0464) -> (277.53, 145.0932) construction
  line L7318 (277.53, 145.0932) -> (277.6833, 145.1411) construction
  line L7319 (277.6833, 145.1411) -> (277.8364, 145.1901) construction
  line L7320 (277.8364, 145.1901) -> (277.9894, 145.2401) construction
  line L7321 (277.9894, 145.2401) -> (278.1423, 145.2913) construction
  line L7322 (278.1423, 145.2913) -> (278.2951, 145.3434) construction
  line L7323 (278.2951, 145.3434) -> (278.4478, 145.3965) construction
  line L7324 (278.4478, 145.3965) -> (278.6003, 145.4507) construction
  line L7325 (278.6003, 145.4507) -> (278.7526, 145.5058) construction
  line L7326 (278.7526, 145.5058) -> (278.9049, 145.562) construction
  line L7327 (278.9049, 145.562) -> (279.057, 145.619) construction
  line L7328 (279.057, 145.619) -> (279.209, 145.6771) construction
  line L7329 (279.209, 145.6771) -> (279.3608, 145.7361) construction
  line L7330 (279.3608, 145.7361) -> (279.5124, 145.7961) construction
  line L7331 (279.5124, 145.7961) -> (279.664, 145.857) construction
  line L7332 (279.664, 145.857) -> (279.8153, 145.9188) construction
  line L7333 (279.8153, 145.9188) -> (279.9665, 145.9815) construction
  line L7334 (279.9665, 145.9815) -> (280.1176, 146.0452) construction
  line L7335 (280.1176, 146.0452) -> (280.2685, 146.1097) construction
  line L7336 (280.2685, 146.1097) -> (280.4192, 146.1751) construction
  line L7337 (280.4192, 146.1751) -> (280.5698, 146.2415) construction
  line L7338 (280.5698, 146.2415) -> (280.7202, 146.3087) construction
  line L7339 (280.7202, 146.3087) -> (280.8704, 146.3767) construction
  line L7340 (280.8704, 146.3767) -> (281.0205, 146.4457) construction
  line L7341 (281.0205, 146.4457) -> (281.1704, 146.5154) construction
  line L7342 (281.1704, 146.5154) -> (281.3201, 146.5861) construction
  line L7343 (281.3201, 146.5861) -> (281.4696, 146.6575) construction
  line L7344 (281.4696, 146.6575) -> (281.619, 146.7299) construction
  line L7345 (281.619, 146.7299) -> (281.7682, 146.803) construction
  line L7346 (281.7682, 146.803) -> (281.9172, 146.877) construction
  line L7347 (281.9172, 146.877) -> (282.066, 146.9518) construction
  line L7348 (282.066, 146.9518) -> (282.2146, 147.0274) construction
  line L7349 (282.2146, 147.0274) -> (282.3631, 147.1038) construction
  line L7350 (282.3631, 147.1038) -> (282.5113, 147.181) construction
  line L7351 (282.5113, 147.181) -> (282.6594, 147.259) construction
  line L7352 (282.6594, 147.259) -> (282.8072, 147.3378) construction
  line L7353 (282.8072, 147.3378) -> (282.9549, 147.4174) construction
  line L7354 (282.9549, 147.4174) -> (283.1023, 147.4977) construction
  line L7355 (283.1023, 147.4977) -> (283.2496, 147.5789) construction
  line L7356 (283.2496, 147.5789) -> (283.3672, 147.6444) construction
  line L7357 (283.3672, 147.6444) -> (283.4554, 147.6939) construction
  line L7358 (283.4554, 147.6939) -> (283.5141, 147.7271) construction
  line L7359 (283.5141, 147.7271) -> (283.5435, 147.7437) construction
  spline S98 degree 5 poles (225.4942, 90.4458) (225.501, 90.4157) (225.5153, 90.3556) (225.5391, 90.2662) (225.5755, 90.1483) (225.6271, 90.0027) (225.6831, 89.8584) (225.7419, 89.7148) (225.8021, 89.5717) (225.8633, 89.4289) (225.9255, 89.2864) (225.9891, 89.1443) (226.0546, 89.0029) (226.1222, 88.8621) (226.192, 88.7221) (226.2636, 88.5827) (226.337, 88.4439) (226.4117, 88.3056) (226.4877, 88.1678) (226.5647, 88.0303) (226.6429, 87.8933) (226.7224, 87.7568) (226.8031, 87.6208) (226.885, 87.4852) (226.9683, 87.3502) (227.0528, 87.2157) (227.1384, 87.0816) (227.2252, 86.948) (227.313, 86.8148) (227.4018, 86.682) (227.4917, 86.5497) (227.5826, 86.4179) (227.6745, 86.2865) (227.7674, 86.1555) (227.8613, 86.025) (227.9562, 85.895) (228.052, 85.7654) (228.1488, 85.6362) (228.2466, 85.5074) (228.3452, 85.3791) (228.4447, 85.2512) (228.5451, 85.1238) (228.6464, 84.9968) (228.7486, 84.8702) (228.8516, 84.744) (228.9555, 84.6183) (229.0603, 84.493) (229.1658, 84.3682) (229.2722, 84.2438) (229.3794, 84.1198) (229.4875, 83.9962) (229.5963, 83.8731) (229.7059, 83.7503) (229.8162, 83.6281) (229.9274, 83.5062) (230.0393, 83.3848) (230.152, 83.2638) (230.2655, 83.1432) (230.3797, 83.0231) (230.4946, 82.9034) (230.6102, 82.7841) (230.7266, 82.6653) (230.8438, 82.5469) (230.9616, 82.4289) (231.0801, 82.3113) (231.1994, 82.1942) (231.3193, 82.0775) (231.4399, 81.9612) (231.5613, 81.8454) (231.6832, 81.73) (231.8059, 81.615) (231.9046, 81.5233) (231.9789, 81.4548) (232.0286, 81.4092) (232.0535, 81.3864) knots 0 0 0 0 0 0 0.01428571 0.02857143 0.04285714 0.05714286 0.07142857 0.08571429 0.1 0.11428571 0.12857143 0.14285714 0.15714286 0.17142857 0.18571429 0.2 0.21428571 0.22857143 0.24285714 0.25714286 0.27142857 0.28571429 0.3 0.31428571 0.32857143 0.34285714 0.35714286 0.37142857 0.38571429 0.4 0.41428571 0.42857143 0.44285714 0.45714286 0.47142857 0.48571429 0.5 0.51428571 0.52857143 0.54285714 0.55714286 0.57142857 0.58571429 0.6 0.61428571 0.62857143 0.64285714 0.65714286 0.67142857 0.68571429 0.7 0.71428571 0.72857143 0.74285714 0.75714286 0.77142857 0.78571429 0.8 0.81428571 0.82857143 0.84285714 0.85714286 0.87142857 0.88571429 0.9 0.91428571 0.92857143 0.94285714 0.95714286 0.97142857 0.98571429 1 1 1 1 1 1
  line L7360 (225.4942, 90.4458) -> (225.501, 90.4157) construction
  line L7361 (225.501, 90.4157) -> (225.5153, 90.3556) construction
  line L7362 (225.5153, 90.3556) -> (225.5391, 90.2662) construction
  line L7363 (225.5391, 90.2662) -> (225.5755, 90.1483) construction
  line L7364 (225.5755, 90.1483) -> (225.6271, 90.0027) construction
  line L7365 (225.6271, 90.0027) -> (225.6831, 89.8584) construction
  line L7366 (225.6831, 89.8584) -> (225.7419, 89.7148) construction
  line L7367 (225.7419, 89.7148) -> (225.8021, 89.5717) construction
  line L7368 (225.8021, 89.5717) -> (225.8633, 89.4289) construction
  line L7369 (225.8633, 89.4289) -> (225.9255, 89.2864) construction
  line L7370 (225.9255, 89.2864) -> (225.9891, 89.1443) construction
  line L7371 (225.9891, 89.1443) -> (226.0546, 89.0029) construction
  line L7372 (226.0546, 89.0029) -> (226.1222, 88.8621) construction
  line L7373 (226.1222, 88.8621) -> (226.192, 88.7221) construction
  line L7374 (226.192, 88.7221) -> (226.2636, 88.5827) construction
  line L7375 (226.2636, 88.5827) -> (226.337, 88.4439) construction
  line L7376 (226.337, 88.4439) -> (226.4117, 88.3056) construction
  line L7377 (226.4117, 88.3056) -> (226.4877, 88.1678) construction
  line L7378 (226.4877, 88.1678) -> (226.5647, 88.0303) construction
  line L7379 (226.5647, 88.0303) -> (226.6429, 87.8933) construction
  line L7380 (226.6429, 87.8933) -> (226.7224, 87.7568) construction
  line L7381 (226.7224, 87.7568) -> (226.8031, 87.6208) construction
  line L7382 (226.8031, 87.6208) -> (226.885, 87.4852) construction
  line L7383 (226.885, 87.4852) -> (226.9683, 87.3502) construction
  line L7384 (226.9683, 87.3502) -> (227.0528, 87.2157) construction
  line L7385 (227.0528, 87.2157) -> (227.1384, 87.0816) construction
  line L7386 (227.1384, 87.0816) -> (227.2252, 86.948) construction
  line L7387 (227.2252, 86.948) -> (227.313, 86.8148) construction
  line L7388 (227.313, 86.8148) -> (227.4018, 86.682) construction
  line L7389 (227.4018, 86.682) -> (227.4917, 86.5497) construction
  line L7390 (227.4917, 86.5497) -> (227.5826, 86.4179) construction
  line L7391 (227.5826, 86.4179) -> (227.6745, 86.2865) construction
  line L7392 (227.6745, 86.2865) -> (227.7674, 86.1555) construction
  line L7393 (227.7674, 86.1555) -> (227.8613, 86.025) construction
  line L7394 (227.8613, 86.025) -> (227.9562, 85.895) construction
  line L7395 (227.9562, 85.895) -> (228.052, 85.7654) construction
  line L7396 (228.052, 85.7654) -> (228.1488, 85.6362) construction
  line L7397 (228.1488, 85.6362) -> (228.2466, 85.5074) construction
  line L7398 (228.2466, 85.5074) -> (228.3452, 85.3791) construction
  line L7399 (228.3452, 85.3791) -> (228.4447, 85.2512) construction
  line L7400 (228.4447, 85.2512) -> (228.5451, 85.1238) construction
  line L7401 (228.5451, 85.1238) -> (228.6464, 84.9968) construction
  line L7402 (228.6464, 84.9968) -> (228.7486, 84.8702) construction
  line L7403 (228.7486, 84.8702) -> (228.8516, 84.744) construction
  line L7404 (228.8516, 84.744) -> (228.9555, 84.6183) construction
  line L7405 (228.9555, 84.6183) -> (229.0603, 84.493) construction
  line L7406 (229.0603, 84.493) -> (229.1658, 84.3682) construction
  line L7407 (229.1658, 84.3682) -> (229.2722, 84.2438) construction
  line L7408 (229.2722, 84.2438) -> (229.3794, 84.1198) construction
  line L7409 (229.3794, 84.1198) -> (229.4875, 83.9962) construction
  line L7410 (229.4875, 83.9962) -> (229.5963, 83.8731) construction
  line L7411 (229.5963, 83.8731) -> (229.7059, 83.7503) construction
  line L7412 (229.7059, 83.7503) -> (229.8162, 83.6281) construction
  line L7413 (229.8162, 83.6281) -> (229.9274, 83.5062) construction
  line L7414 (229.9274, 83.5062) -> (230.0393, 83.3848) construction
  line L7415 (230.0393, 83.3848) -> (230.152, 83.2638) construction
  line L7416 (230.152, 83.2638) -> (230.2655, 83.1432) construction
  line L7417 (230.2655, 83.1432) -> (230.3797, 83.0231) construction
  line L7418 (230.3797, 83.0231) -> (230.4946, 82.9034) construction
  line L7419 (230.4946, 82.9034) -> (230.6102, 82.7841) construction
  line L7420 (230.6102, 82.7841) -> (230.7266, 82.6653) construction
  line L7421 (230.7266, 82.6653) -> (230.8438, 82.5469) construction
  line L7422 (230.8438, 82.5469) -> (230.9616, 82.4289) construction
  line L7423 (230.9616, 82.4289) -> (231.0801, 82.3113) construction
  line L7424 (231.0801, 82.3113) -> (231.1994, 82.1942) construction
  line L7425 (231.1994, 82.1942) -> (231.3193, 82.0775) construction
  line L7426 (231.3193, 82.0775) -> (231.4399, 81.9612) construction
  line L7427 (231.4399, 81.9612) -> (231.5613, 81.8454) construction
  line L7428 (231.5613, 81.8454) -> (231.6832, 81.73) construction
  line L7429 (231.6832, 81.73) -> (231.8059, 81.615) construction
  line L7430 (231.8059, 81.615) -> (231.9046, 81.5233) construction
  line L7431 (231.9046, 81.5233) -> (231.9789, 81.4548) construction
  line L7432 (231.9789, 81.4548) -> (232.0286, 81.4092) construction
  line L7433 (232.0286, 81.4092) -> (232.0535, 81.3864) construction
  arc A188 (187.6019, 201.9354) -> (184.5338, 200.3721) centre (212.132, 150) ccw